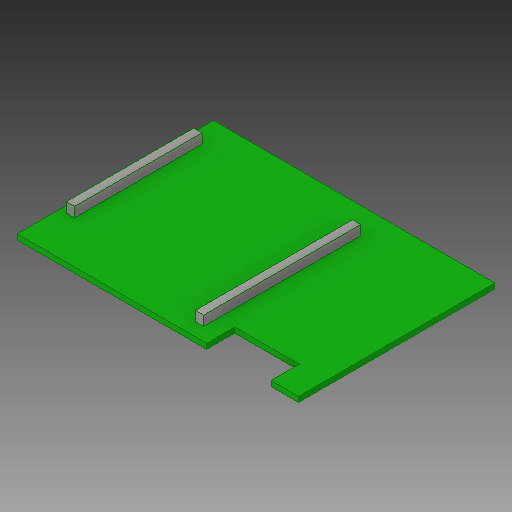
# Autodesk Inventor part: PCB Wifi
Saved by Autodesk Inventor 2019 (Build 230136000, 136)
## iProperties
Created: 2018-06-11
Part Number: PCB Wifi
Material: Nylon, disulfure de molybdène
Document SubType Name: Modeling
Designer: dimercur
Density: 1.13 g/cm^3
Appearance: Vert foncé
Mass: 8.39635 g
Surface Area: 97.36 cm^2
Volume: 7.4304 cm^3
Author: dimercur
Autodesk Inventor part; units mm, degrees
ref_plane "YZ Plane" through (0, 0, 0) normal (1, 0, 0) x (0, 1, 0)
ref_plane "XZ Plane" through (0, 0, 0) normal (0, 1, 0) x (-1, 0, 0)
ref_plane "XY Plane" through (0, 0, 0) normal (0, 0, 1) x (1, 0, 0)
sketch "Esquisse1" plane through (0, 0, 0) normal (0, 1, 0) x (-1, 0, 0)
  line L0 (43, -30) -> (-43, -30)
  line L1 (-43, -30) -> (-43, 30)
  line L2 (-43, 30) -> (43, 30)
  line L3 (43, 30) -> (43, -30)
  point P0 (0, 0)
  dimension "d0" = 86
  dimension "d1" = 43
  dimension "d2" = 60
  dimension "d3" = 30
  constraints: 8 end point, 2 parallel, 1 horizontal, 1 perpendicular
  measures "d0" distance of L0.start L0.end
  measures "d1" horizontal distance of point (0, 0) L0.start
  measures "d2" distance of L2.end L0.start
  measures "d3" vertical distance of point (0, 0) L0.start
extrude "Extrusion1" add sketch "Esquisse1" along normal blind 1.6
sketch "Esquisse2" plane through (0, 1.6, 0) normal (0, 1, 0) x (1, 0, 0)
  line L0 (-41, 22) -> (-38.5, 22)
  line L1 (-38.5, 22) -> (-38.5, -17)
  line L2 (-38.5, -17) -> (-41, -17)
  line L3 (-41, -17) -> (-41, 22)
  line L4 (7.5, 22) -> (10, 22)
  line L5 (10, 22) -> (10, -26)
  line L6 (10, -26) -> (7.5, -26)
  line L7 (7.5, -26) -> (7.5, 22)
  line L8 (43, 30) -> (-43, 30) projected
  line L9 (-43, 30) -> (-43, -30) projected
  point P0 (0, 0)
  dimension "d6" = 2.5
  dimension "d7" = 2.5
  dimension "d8" = 39
  dimension "d9" = 48
  dimension "d10" = 8
  dimension "d11" = 2
  dimension "d12" = 46
  constraints: 16 end point, 4 parallel, 2 horizontal, 2 perpendicular, 1 point on line
  measures "d6" distance of L0.start L0.end
  measures "d7" distance of L4.start L4.end
  measures "d8" distance of L2.end L0.start
  measures "d9" distance of L6.end L4.start
  measures "d10" distance between parallel lines of L8 L0
  measures "d11" distance between parallel lines of L9 L3
  measures "d12" distance between parallel lines of L7 L1
extrude "Extrusion2" add sketch "Esquisse2" along normal blind 3
sketch "Esquisse3" plane through (0, 0, 0) normal (0, -1, 0) x (1, 0, 0)
  line L0 (43, 30) -> (-43, 30) projected
  line L1 (14.9, 30) -> (34.6, 30)
  line L2 (34.6, 30) -> (34.6, 21.4)
  line L3 (34.6, 21.4) -> (14.9, 21.4)
  line L4 (14.9, 21.4) -> (14.9, 30)
  line L5 (43, -30) -> (43, 30) projected
  point P0 (0, 0)
  dimension "d15" = 8.4
  dimension "d16" = 28.1
  dimension "d17" = 8.6
  constraints: 8 end point, 2 parallel, 1 horizontal, 1 perpendicular, 1 point on line
  measures "d15" distance between parallel lines of L5 L2
  measures "d16" distance between parallel lines of L5 L4
  measures "d17" distance of L1.end L2.end
extrude "Extrusion3" cut sketch "Esquisse3" against normal through all
sketch "Esquisse4" plane through (0, 0, 0) normal (0, -1, 0) x (1, 0, 0)
  line L0 (40, -11) -> (37.5, -11)
  line L1 (37.5, -11) -> (37.5, 28)
  line L2 (37.5, 28) -> (40, 28)
  line L3 (40, 28) -> (40, -11)
  line L4 (-11, -20) -> (-11, 28)
  line L5 (-11, 28) -> (-8.5, 28)
  line L6 (-8.5, 28) -> (-8.5, -20)
  line L7 (43, -30) -> (43, 30) projected
  line L8 (43, 30) -> (34.6, 30) projected
  line L9 (-43, -30) -> (43, -30) projected
  line L10 (-43, 30) -> (-43, -30) projected
  line L11 (-8.5, -20) -> (-11, -20)
  line L12 (14.9, 30) -> (-43, 30) projected
  point P0 (0, 0)
  point P1 (43, -25.5)
  point P2 (43, 25.5)
  point P3 (41.5, 27)
  point P4 (36.1, 27)
  point P5 (-41.5, -27)
  point P6 (41.5, -27)
  point P7 (34.6, 30)
  dimension "d21" = 39
  dimension "d22" = 48
  dimension "d23" = 2.5
  dimension "d24" = 2.5
  dimension "d25" = 46
  dimension "d32" = 32
  dimension "d37" = 2
  dimension "d38" = 2
  constraints: 16 end point, 3 parallel, 2 horizontal, 1 perpendicular, 2 other
  measures "d21" distance of L2.end L0.start
  measures "d22" distance of L4.start L4.end
  measures "d23" distance of L0.start L0.end
  measures "d24" distance of L6.end L4.start
  measures "d25" distance between parallel lines of L6 L1
  measures "d32" distance between parallel lines of L10 L4
  measures "d37" distance between parallel lines of L12 L5
  measures "d38" distance between parallel lines of L12 L2
extrude "Extrusion4" add sketch "Esquisse4" along normal blind 0.1
equation "\"d1\" = 0.5 * d0"
equation "\"d3\" = 0.5 * d2"
equation "\"d24\" = d23"
equation "\"d38\" = d37"
